Autodesk Inventor part; units mm, degrees
(part 2 of 2)
  line L291 (76.6309, -51.1711) -> (76.9782, -53.1407)
  line L292 (88.4022, -66.9949) -> (87.1522, -64.8299)
  line L293 (87.1522, -64.8299) -> (93.4363, -53.9456)
  line L294 (81.9782, -70.4613) -> (86.9022, -69.593)
  line L295 (86.9022, -69.593) -> (88.4022, -66.9949)
  line L296 (74.4782, -57.4709) -> (81.9782, -70.4613)
  line L297 (82.6309, -40.7789) -> (83.6309, -39.0468) construction
  line L298 (82.6309, -40.7789) -> (84.5103, -40.0949)
  line L299 (79.6309, -45.975) -> (82.6309, -40.7789)
  line L300 (84.5103, -40.0949) -> (87.0103, -35.7647)
  line L301 (87.0103, -35.7647) -> (102.0103, -35.7647)
  line L302 (103.7204, -40.4632) -> (102.2204, -43.0613)
  line L303 (102.2204, -43.0613) -> (99.7204, -43.0613)
  line L304 (102.0103, -35.7647) -> (103.7204, -40.4632)
  line L305 (99.7204, -43.0613) -> (93.4363, -53.9456)
  line L306 (79.6309, 45.9748) -> (82.6309, 40.7787)
  line L307 (84.5103, 40.0947) -> (87.0103, 35.7646)
  line L308 (82.6309, 40.7787) -> (84.5103, 40.0947)
  line L309 (102.2204, 43.0611) -> (99.7204, 43.0611)
  line L310 (99.7204, 43.0611) -> (93.4363, 53.9454)
  line L311 (102.0103, 35.7646) -> (103.7204, 40.463)
  line L312 (103.7204, 40.463) -> (102.2204, 43.0611)
  line L313 (87.0103, 35.7646) -> (102.0103, 35.7646)
  line L314 (76.6309, 51.171) -> (75.6309, 52.903) construction
  line L315 (76.6309, 51.171) -> (76.9782, 53.1406)
  line L316 (79.6309, 45.9748) -> (76.6309, 51.171)
  line L317 (76.9782, 53.1406) -> (74.4782, 57.4707)
  line L318 (74.4782, 57.4707) -> (81.9782, 70.4611)
  line L319 (86.9022, 69.5928) -> (88.4022, 66.9948)
  line L320 (88.4022, 66.9948) -> (87.1522, 64.8297)
  line L321 (81.9782, 70.4611) -> (86.9022, 69.5928)
  line L322 (87.1522, 64.8297) -> (93.4363, 53.9454)
  line L323 (0, 91.9498) -> (5.9999, 91.9498)
  line L324 (7.532, 93.2354) -> (12.532, 93.2354)
  line L325 (5.9999, 91.9498) -> (7.532, 93.2354)
  line L326 (13.8181, 110.056) -> (12.5681, 107.8909)
  line L327 (12.5681, 107.8909) -> (0, 107.8909)
  line L328 (20.032, 106.2257) -> (16.8181, 110.056)
  line L329 (16.8181, 110.056) -> (13.8181, 110.056)
  line L330 (12.532, 93.2354) -> (20.032, 106.2257)
  line L331 (-6, 91.9498) -> (-8, 91.9498) construction
  line L332 (-6, 91.9498) -> (-7.5321, 93.2354)
  line L333 (0, 91.9498) -> (-6, 91.9498)
  line L334 (-7.5321, 93.2354) -> (-12.5321, 93.2354)
  line L335 (-12.5321, 93.2354) -> (-20.0321, 106.2257)
  line L336 (-16.8181, 110.056) -> (-13.8181, 110.056)
  line L337 (-13.8181, 110.056) -> (-12.5681, 107.8909)
  line L338 (-20.0321, 106.2257) -> (-16.8181, 110.056)
  line L339 (-12.5681, 107.8909) -> (0, 107.8909)
  line L340 (-79.6309, 45.9748) -> (-76.631, 51.171)
  line L341 (-76.9783, 53.1406) -> (-74.4783, 57.4707)
  line L342 (-76.631, 51.171) -> (-76.9783, 53.1406)
  line L343 (-88.4023, 66.9948) -> (-87.1523, 64.8297)
  line L344 (-87.1523, 64.8297) -> (-93.4364, 53.9454)
  line L345 (-81.9783, 70.4611) -> (-86.9023, 69.5928)
  line L346 (-86.9023, 69.5928) -> (-88.4023, 66.9948)
  line L347 (-74.4783, 57.4707) -> (-81.9783, 70.4611)
  line L348 (-82.6309, 40.7787) -> (-83.6309, 39.0467) construction
  line L349 (-82.6309, 40.7787) -> (-84.5103, 40.0947)
  line L350 (-79.6309, 45.9748) -> (-82.6309, 40.7787)
  line L351 (-84.5103, 40.0947) -> (-87.0103, 35.7646)
  line L352 (-87.0103, 35.7646) -> (-102.0103, 35.7646)
  line L353 (-103.7204, 40.463) -> (-102.2204, 43.0611)
  line L354 (-102.2204, 43.0611) -> (-99.7204, 43.0611)
  line L355 (-102.0103, 35.7646) -> (-103.7204, 40.463)
  line L356 (-99.7204, 43.0611) -> (-93.4364, 53.9454)
  line L357 (-79.6309, -45.975) -> (-82.6309, -40.7789)
  line L358 (-84.5103, -40.0949) -> (-87.0103, -35.7647)
  line L359 (-82.6309, -40.7789) -> (-84.5103, -40.0949)
  line L360 (-102.2204, -43.0613) -> (-99.7204, -43.0613)
  line L361 (-99.7204, -43.0613) -> (-93.4364, -53.9456)
  line L362 (-102.0103, -35.7647) -> (-103.7204, -40.4632)
  line L363 (-103.7204, -40.4632) -> (-102.2204, -43.0613)
  line L364 (-87.0103, -35.7647) -> (-102.0103, -35.7647)
  line L365 (-76.631, -51.1711) -> (-75.631, -52.9032) construction
  line L366 (-76.631, -51.1711) -> (-76.9783, -53.1407)
  line L367 (-79.6309, -45.975) -> (-76.631, -51.1711)
  line L368 (-76.9783, -53.1407) -> (-74.4783, -57.4709)
  line L369 (-74.4783, -57.4709) -> (-81.9783, -70.4613)
  line L370 (-86.9023, -69.593) -> (-88.4023, -66.9949)
  line L371 (-88.4023, -66.9949) -> (-87.1523, -64.8299)
  line L372 (-81.9783, -70.4613) -> (-86.9023, -69.593)
  line L373 (-87.1523, -64.8299) -> (-93.4364, -53.9456)
  line L374 (0, -138) -> (0, -141)
  line L375 (0, -138) -> (3, -138) construction
  line L376 (-25, -138) -> (-22, -138) construction
  line L377 (-25, -138) -> (-20, -138) construction
  line L378 (0, -141) -> (-27.5173, -141)
  line L379 (0, -141) -> (27.5173, -141) construction
  line L380 (-27.5173, -141) -> (-13.8071, -141) construction
  line L381 (-28.4202, -128.6031) -> (-34.2721, -128.6031)
  line L382 (-28.4202, -128.6031) -> (-22.5683, -128.6031) construction
  line L383 (-107.0114, -90.6507) -> (-104.0114, -90.6507) construction
  line L384 (-27.5173, -141) -> (-30.9375, -131.6031)
  line L385 (-27.5173, -141) -> (-17.5173, -141) construction
  line L386 (0, -141) -> (27.5173, -141)
  line L387 (27.5173, -141) -> (13.8071, -141) construction
  line L388 (27.5173, -141) -> (30.9375, -131.6031)
  line L389 (108.3508, -94.3307) -> (98.5028, -92.5942)
  line L390 (122.1095, -70.5) -> (108.3508, -94.3307)
  line L391 (122.1095, -70.5) -> (135.8681, -46.6693) construction
  line L392 (122.1095, -70.5) -> (135.8681, -46.6693)
  line L393 (135.8681, -46.6693) -> (129.4403, -39.0089)
  line L394 (135.8681, 46.6692) -> (129.4402, 39.0088)
  line L395 (122.1095, 70.4999) -> (135.8681, 46.6692)
  line L396 (122.1095, 70.4999) -> (108.3508, 94.3306) construction
  line L397 (122.1095, 70.4999) -> (108.3508, 94.3306)
  line L398 (108.3508, 94.3306) -> (98.5027, 92.5941)
  line L399 (27.5172, 140.9998) -> (30.9374, 131.6029)
  line L400 (-0.0001, 140.9998) -> (27.5172, 140.9998)
  line L401 (-0.0001, 140.9998) -> (-27.5173, 140.9998) construction
  line L402 (-0.0001, 140.9998) -> (-27.5173, 140.9998)
  line L403 (-27.5173, 140.9998) -> (-30.9376, 131.6029)
  line L404 (-108.3509, 94.3305) -> (-98.5028, 92.5941)
  line L405 (-122.1095, 70.4999) -> (-108.3509, 94.3305)
  line L406 (-122.1095, 70.4999) -> (-135.8682, 46.6692) construction
  line L407 (-122.1095, 70.4999) -> (-135.8682, 46.6692)
  line L408 (-135.8682, 46.6692) -> (-129.4403, 39.0087)
  line L409 (-135.8682, -46.6694) -> (-129.4403, -39.0089)
  line L410 (-122.1095, -70.5001) -> (-135.8682, -46.6694)
  line L411 (-122.1095, -70.5001) -> (-108.3509, -94.3307) construction
  line L412 (-122.1095, -70.5001) -> (-108.3509, -94.3307)
  line L413 (-108.3509, -94.3307) -> (-98.5028, -92.5943)
  line L414 (-30.9375, -131.6031) -> (-98.5028, -92.5943)
  line L415 (98.5028, -92.5942) -> (30.9375, -131.6031)
  line L416 (129.4402, 39.0088) -> (129.4403, -39.0089)
  line L417 (30.9374, 131.6029) -> (98.5027, 92.5941)
  line L418 (-98.5028, 92.5941) -> (-30.9376, 131.6029)
  line L419 (-129.4403, -39.0089) -> (-129.4403, 39.0087)
  point P0 (0, 0)
  point P1 (0, -0.0001)
  point P2 (-50.3385, -87.1889)
  point P3 (-50.3385, -87.1889)
  point P4 (-50.3385, -87.1889)
  point P5 (-50.3385, -87.1889)
  point P6 (-50.3385, -87.1889)
  point P7 (28.4201, -128.6031)
  point P8 (-28.4202, 128.6029)
  point P9 (129.4403, -39.0089)
  point P10 (28.4201, -128.6031)
  dimension "d759" = 3.2
  dimension "d760" = 3.2
  dimension "d761" = 10.5
  dimension "d762" = 3
  dimension "d763" = 10.5
  dimension "d764" = 10.5
  dimension "d765" = 10.5
  dimension "d766" = 3
  dimension "d767" = 3
  dimension "d768" = 3
  dimension "d769" = 30
  dimension "d770" = 30
  dimension "d771" = 30
  dimension "d772" = 30
  dimension "d773" = 120
  dimension "d774" = 25
  dimension "d775" = 30
  dimension "d776" = 25
  dimension "d777" = 150
  dimension "d778" = 0
  dimension "d779" = 180
  dimension "d780" = 10
  dimension "d781" = 110
  dimension "d782" = 360
  dimension "d783" = 360
  dimension "d784" = 3.3
  dimension "d785" = 3.3
  dimension "d786" = 360
  dimension "d787" = 30
  dimension "d788" = 30
  dimension "d789" = 10.9
  dimension "d790" = 90
  dimension "d791" = 12.76
  dimension "d792" = 120
  dimension "d793" = 8.7
  dimension "d794" = 90
  dimension "d795" = 10.534
  dimension "d796" = 130
  dimension "d797" = 10.5
  dimension "d798" = 3
  dimension "d799" = 130
  dimension "d800" = 52.528
  dimension "d801" = 6
  dimension "d802" = 2.5
  dimension "d803" = 40
  dimension "d804" = 7
  dimension "d805" = 20
  dimension "d806" = 60
  dimension "d807" = 9
  dimension "d808" = 129.999
  dimension "d809" = 180
  dimension "d810" = 4.5
  dimension "d811" = 120
  dimension "d812" = 360
  dimension "d813" = 3
  dimension "d814" = 2
  dimension "d815" = 40
  dimension "d816" = 5
  dimension "d817" = 140
  dimension "d818" = 15
  dimension "d819" = 120
  dimension "d820" = 5
  dimension "d821" = 110
  dimension "d822" = 3
  constraints: 840 end point, 40 horizontal, 35 centre point, 20 equal length, 10 symmetric about line, 3 parallel, 3 vertical, 2 coincident, 2 perpendicular, 787 other
  measures "d759" diameter of A0
  measures "d760" diameter of A1
  measures "d761" distance of L0.end L0.start
  measures "d762" diameter of A2
  measures "d763" distance of L1.start L1.end
  measures "d764" distance of L1.start L2.end
  measures "d765" distance of L1.start L3.end
  measures "d766" diameter of A3
  measures "d767" diameter of A4
  measures "d768" diameter of A5
  measures "d769" distance of L4.start L4.end
  measures "d770" distance of L5.start L5.end
  measures "d771" distance of L6.start L6.end
  measures "d772" distance of L7.start L7.end
  measures "d773" angle of L7 L8
  measures "d774" distance of L10.start L10.end
  measures "d775" angle of L10 L11
  measures "d776" distance of L12.start L12.end
  measures "d777" angle of L12 L13
  measures "d778" distance between parallel lines of L15 L16
  measures "d779" angle of L17 L18
  measures "d780" distance of L17.end L24.end
  measures "d781" angle of L25 L24
  measures "d784" diameter of A23
  measures "d785" diameter of A24
  measures "d787" distance of point (0, 0) L81.start
  measures "d788" distance of point (0, 0) L79.start
  measures "d789" distance of L79.start L79.end
  measures "d790" angle of L79 L80
  measures "d791" distance of L79.end L82.end
  measures "d792" angle of L82 L83
  measures "d793" distance of L82.end L84.end
  measures "d794" angle of L84 L85
  measures "d795" distance of L84.end L86.end
  measures "d796" angle of L86 L87
  measures "d797" distance of L86.end L88.end
  measures "d798" distance of L88.end L89.end
  measures "d799" angle of L90 L89
  measures "d800" distance of L90.end L113.start
  measures "d801" distance of L113.start L113.end
  measures "d802" distance of L113.end L115.end
  measures "d803" angle of L115 L116
  measures "d804" distance of L115.end L117.end
  measures "d805" distance of L117.end L118.end
  measures "d806" angle of L118 L119
  measures "d807" distance of L118.end L120.end
  measures "d808" angle of L120 L121
  measures "d809" angle of L122 L123
  measures "d810" distance of L122.end L124.end
  measures "d811" angle of L125 L124
  measures "d813" distance of L113.start L271.start
  measures "d814" distance of L271.end L272.end
  measures "d815" angle of L272 L273
  measures "d816" distance of L272.end L274.end
  measures "d817" angle of L274 L272
  measures "d818" distance of L274.end L275.end
  measures "d819" angle of L274 L275
  measures "d820" distance of L275.end L276.end
  measures "d821" angle of L275 L276
  measures "d822" distance of L276.end L277.end
extrude "Extrusion12" add sketch "Sketch3" against normal blind 3 separate body contours L164 L162 L165 L157 L155 L158 L160 L140 L10 L305 L303 L302 L304 L301 L300 L298 L299 | L10 L289 L291 L290 L296 L294 L295 L292 L293 L141 L142 L147 L146 L148 L153 L152 L149 | L268 L266 L269 L261 L259 L262 L264 L244 L12 L373 L371 L370 L372 L369 L368 L366 L367 | L12 L357 L359 L358 L364 L362 L363 L360 L361 L245 L246 L251 L250 L252 L257 L256 L253 | L113 L115 L117 L118 L120 L122 L124 L126 L127 L139 L129 L136 L137 L134 L131 L130 | L166 L167 L168 L173 L172 L174 L179 L178 L175 L190 L188 L191 L183 L181 L184 L186 | L192 L193 L194 L199 L198 L200 L205 L204 L201 L216 L214 L217 L209 L207 L210 L212 | L218 L219 L220 L225 L224 L226 L231 L230 L227 L242 L240 L243 L235 L233 L236 L238 | L378 L384 L414 L413 L412 L410 L409 L419 L408 L407 L405 L404 L418 L403 L402 L400 L399 L417 L398 L397 L395 L394 L416 L393 L392 L390 L389 L415 L388 L386
fillet "Fillet12" radius 5 24 edges at (-98.5028, 1.5, 92.5943) (-108.3509, 1.5, 94.3307) (-135.8682, 1.5, 46.6694) (-129.4403, 1.5, 39.0089) (-129.4403, 1.5, -39.0087) (-135.8682, 1.5, -46.6692) (-108.3509, 1.5, -94.3305) (-98.5028, 1.5, -92.5941) (-30.9376, 1.5, -131.6029) (-27.5173, 1.5, -140.9998) (27.5172, 1.5, -140.9998) (30.9374, 1.5, -131.6029) (98.5027, 1.5, -92.5941) (108.3508, 1.5, -94.3306) (135.8681, 1.5, -46.6692) (129.4402, 1.5, -39.0088) (129.4403, 1.5, 39.0089) (135.8681, 1.5, 46.6693) (108.3508, 1.5, 94.3307) (98.5028, 1.5, 92.5942) (30.9375, 1.5, 131.6031) (27.5173, 1.5, 141) (-27.5173, 1.5, 141) (-30.9375, 1.5, 131.6031)
fillet "Fillet13" radius 2 108 edges at (-30.2097, 1.5, -30.6505) (-23.4386, 1.5, -38.72) (-12.9386, 1.5, -38.72) (-11.0102, 1.5, -36.4219) (11.0102, 1.5, -36.4219) (12.9386, 1.5, -38.72) (23.4386, 1.5, -38.72) (30.2097, 1.5, -30.6505) (30.2097, 1.5, -21.9505) (36.5897, 1.5, -10.9001) (36.5897, 1.5, 10.8999) (30.2097, 1.5, 21.9504) (30.2097, 1.5, 30.6504) (23.4386, 1.5, 38.7199) (12.9386, 1.5, 38.7199) (11.0102, 1.5, 36.4218) (-11.0102, 1.5, 36.4218) (-12.9386, 1.5, 38.7199) (-23.4386, 1.5, 38.7199) (-30.2097, 1.5, 30.6504) (-30.2097, 1.5, 21.9504) (-36.5897, 1.5, 10.8999) (-36.5897, 1.5, -10.9001) (-30.2097, 1.5, -21.9505) (-76.9783, 1.5, -53.1406) (-76.631, 1.5, -51.171) (-82.6309, 1.5, -40.7787) (-84.5103, 1.5, -40.0947) (-87.0103, 1.5, -35.7646) (-102.0103, 1.5, -35.7646) (-103.7204, 1.5, -40.463) (-102.2204, 1.5, -43.0611) (-99.7204, 1.5, -43.0611) (-86.9023, 1.5, -69.5928) (-81.9783, 1.5, -70.4611) (-74.4783, 1.5, -57.4707) (-87.1523, 1.5, -64.8297) (-88.4023, 1.5, -66.9948) (-16.8181, 1.5, -110.056) (-20.0321, 1.5, -106.2257) (-12.5321, 1.5, -93.2354) (-7.5321, 1.5, -93.2354) (-6, 1.5, -91.9498) (-13.8181, 1.5, -110.056) (-12.5681, 1.5, -107.8909) (5.9999, 1.5, -91.9498) (7.532, 1.5, -93.2354) (12.532, 1.5, -93.2354) (12.5681, 1.5, -107.8909) (13.8181, 1.5, -110.056) (16.8181, 1.5, -110.056) (20.032, 1.5, -106.2257) (81.9782, 1.5, -70.4611) (74.4782, 1.5, -57.4707) (76.9782, 1.5, -53.1406) (76.6309, 1.5, -51.171) (82.6309, 1.5, -40.7787) (84.5103, 1.5, -40.0947) (87.0103, 1.5, -35.7646) (102.0103, 1.5, -35.7646) (88.4022, 1.5, -66.9948) (87.1522, 1.5, -64.8297) (86.9022, 1.5, -69.5928) (99.7204, 1.5, -43.0611) (102.2204, 1.5, -43.0611) (103.7204, 1.5, -40.463) (102.2204, 1.5, 43.0613) (99.7204, 1.5, 43.0613) (103.7204, 1.5, 40.4632) (87.1522, 1.5, 64.8299) (88.4022, 1.5, 66.9949) (86.9022, 1.5, 69.593) (81.9782, 1.5, 70.4613) (74.4782, 1.5, 57.4709) (76.9782, 1.5, 53.1407) (76.6309, 1.5, 51.1711) (82.6309, 1.5, 40.7789) (84.5103, 1.5, 40.0949) (87.0103, 1.5, 35.7647) (102.0103, 1.5, 35.7647) (5.9999, 1.5, 91.9499) (7.532, 1.5, 93.2355) (12.532, 1.5, 93.2355) (-6, 1.5, 91.9499) (-7.5321, 1.5, 93.2355) (-12.5321, 1.5, 93.2355) (-20.0321, 1.5, 106.2259) (-16.8181, 1.5, 110.0561) (-13.8181, 1.5, 110.0561) (-12.5681, 1.5, 107.8911) (12.5681, 1.5, 107.8911) (13.8181, 1.5, 110.0561) (16.8181, 1.5, 110.0561) (20.032, 1.5, 106.2259) (-76.631, 1.5, 51.1711) (-76.9783, 1.5, 53.1407) (-74.4783, 1.5, 57.4709) (-81.9783, 1.5, 70.4613) (-86.9023, 1.5, 69.593) (-88.4023, 1.5, 66.9949) (-87.1523, 1.5, 64.8299) (-102.2204, 1.5, 43.0613) (-99.7204, 1.5, 43.0613) (-103.7204, 1.5, 40.4632) (-102.0103, 1.5, 35.7647) (-87.0103, 1.5, 35.7647) (-84.5103, 1.5, 40.0949) (-82.6309, 1.5, 40.7789)
body "Solid11"
body "Solid12"
